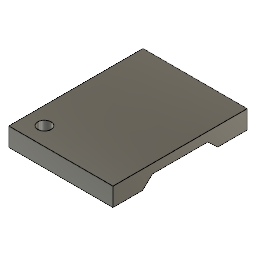
6.5 rectangular pattern (Autodesk Fusion 360 design; units mm, degrees)
Autodesk Fusion 360 part; units mm, degrees
sketch "Sketch1" plane through (0, 0, 0) normal (1, 0, 0) x (0, 1, 0)
  line L0 (0, 0) -> (0, 14.3282)
  line L1 (0, 14.3282) -> (103.0489, 14.3282)
  line L2 (103.0489, 14.3282) -> (103.0489, 0)
  line L3 (51.5244, 0) -> (51.5244, 7.1641) construction
  line L4 (51.5244, 7.1641) -> (72.6846, 7.1641)
  line L5 (72.6846, 7.1641) -> (80.2757, 0)
  line L6 (51.5244, 7.1641) -> (30.3643, 7.1641)
  line L7 (30.3643, 7.1641) -> (22.7732, 0)
  line L8 (103.0489, 0) -> (80.2757, 0)
  line L9 (22.7732, 0) -> (0, 0)
  constraint coincident L0.start L9.end
  constraint vertical L0
  constraint perpendicular L0 L1
  constraint perpendicular L1 L2
  constraint perpendicular L0 L8
  constraint perpendicular L3 L8
  constraint perpendicular L3 L4
  constraint symmetric L4.start L3 L6.start
  constraint symmetric L3 L4.end L6.end
  constraint symmetric L3 L5.end L7.end
  constraint collinear L8 L9
extrude "Extrude1" add sketch "Sketch1" along normal blind 80
sketch "Sketch2" plane through (0, 0, 14.3282) normal (0, 0, 1) x (-1, 0, 0)
  circle A0 centre (-13.5834, -13.8842) radius 5.0923
extrude "Extrude2" cut sketch "Sketch2" against normal through all
